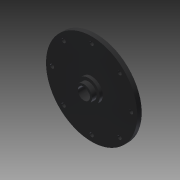
# Autodesk Inventor part: servo arm TGY-S4505B round large
Saved by Autodesk Inventor 2013 (Build 170138000, 138)
## iProperties
Created: 2014-10-08
Part Number: servo arm TGY-S4505B round large
Material: Generic
Document SubType Name: Modeling
Designer: Masta
Density: 1 g/cm^3
Author: Masta
Autodesk Inventor part; units mm, degrees
ref_plane "YZ Plane" through (0, 0, 0) normal (1, 0, 0) x (0, 1, 0)
ref_plane "XZ Plane" through (0, 0, 0) normal (0, 1, 0) x (-1, 0, 0)
ref_plane "XY Plane" through (0, 0, 0) normal (0, 0, 1) x (1, 0, 0)
sketch "Sketch1" plane through (0, 0, 0) normal (0, 1, 0) x (-1, 0, 0)
  circle A0 centre (0, 0) radius 4
  circle A1 centre (0, 0) radius 5.5
  circle A2 centre (0, 0) radius 22.5
  line L0 (0, 0) -> (-19.5, 0) construction
  dimension "d0" = 8
  dimension "d1" = 11
  dimension "d2" = 45
  dimension "d3" = 19.5
  constraints: 4 coincident, 3 centre point, 2 end point, 1 horizontal
  measures "d0" diameter of A0
  measures "d1" diameter of A1
  measures "d2" diameter of A2
  measures "d3" distance of L0.start L0.end
extrude "Extrusion1" add sketch "Sketch1" along normal blind 2.2 contours A0 | A1 | A2
extrude "Extrusion2" add sketch "Sketch1" against normal blind 3.8 contours A0
extrude "Extrusion3" add sketch "Sketch1" against normal blind 1.5 contours A1
hole "Hole1" at (19.5, 0, 0) direction (0, 1, 0) diameter 2 end through all
hole "Hole2" at (0, -3.8, 0) direction (0, 1, 0) diameter 3 end through all
hole "Hole3" at (0, -3.8, 0) direction (0, 1, 0) diameter 6 depth 4
hole "Hole4" at (0, 2.2, 0) direction (0, -1, 0) diameter 6 depth 1
pattern_circular "Circular Pattern1" count 8 over 360 about axis through (0, -10, 0) along (0, 1, 0) of "Hole1"
body "Solid1"
